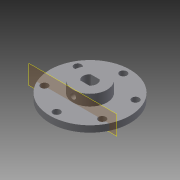
# Autodesk Inventor part: Snowblower Hub
Saved by Autodesk Inventor 2014 (Build 180170000, 170)
## iProperties
Created: 2014-01-06
Part Number: Snowblower Hub
Material: Generic
Document SubType Name: Modeling
Designer: Andrew Toennies
Density: 1 g/cm^3
Appearance: Default
Author: Andrew Toennies
Autodesk Inventor part; units mm, degrees
ref_plane "YZ Plane" through (0, 0, 0) normal (1, 0, 0) x (0, 1, 0)
ref_plane "XZ Plane" through (0, 0, 0) normal (0, 1, 0) x (-1, 0, 0)
ref_plane "XY Plane" through (0, 0, 0) normal (0, 0, 1) x (1, 0, 0)
sketch "Sketch1" plane through (0, 0, 0) normal (0, 1, 0) x (-1, 0, 0)
  circle A0 centre (0, 0) radius 28.575
  dimension "d0" = 57.15
  constraints: 1 centre point, 1 coincident
  measures "d0" diameter of A0
extrude "Extrusion1" add sketch "Sketch1" along normal blind 4.572
sketch "Sketch2" plane through (0, 4.572, 0) normal (0, 1, 0) x (1, 0, 0)
  circle A0 centre (0, 0) radius 28.575 projected
  circle A1 centre (0, 0) radius 12.1666
  dimension "d3" = 24.3332
  constraints: 1 centre point, 1 coincident
  measures "d3" diameter of A1
extrude "Extrusion2" add sketch "Sketch2" along normal blind 7.874 contours A1
sketch "Sketch3" plane through (0, 4.572, 0) normal (0, 1, 0) x (1, 0, 0)
  circle A0 centre (0, 0) radius 28.575 projected
  circle A1 centre (0, 0) radius 23.8125 construction
  circle A2 centre (0, 23.8125) radius 2.5908
  line L0 (0, 0) -> (0, 23.8125) construction
  circle A3 centre (-20.6222, 11.9063) radius 2.5908
  circle A4 centre (-20.6222, -11.9062) radius 2.5908
  circle A5 centre (0, -23.8125) radius 2.5908
  circle A6 centre (20.6222, -11.9063) radius 2.5908
  circle A7 centre (20.6222, 11.9062) radius 2.5908
  dimension "d6" = 47.625
  dimension "d7" = 5.1816
  dimension "d10" = 360
  constraints: 6 centre point, 2 end point, 1 coincident, 1 vertical, 1 vertical alignment, 15 other
  measures "d7" diameter of A2
extrude "Extrusion3" cut sketch "Sketch3" against normal blind 7.874 contours A2 | A3 | A4 | A5 | A6 | A7
sketch "Sketch4" plane through (0, 12.446, 0) normal (0, 1, 0) x (1, 0, 0)
  circle A0 centre (0, 0) radius 12.1666 projected
  line L0 (-3.304, 3.7529) -> (3.304, 3.7529)
  line L1 (-3.304, -3.7528) -> (3.304, -3.7528)
  line L2 (3.304, 3.7529) -> (3.304, -3.7528) construction
  line L3 (-3.304, 3.7529) -> (-3.304, -3.7528) construction
  arc A1 (-3.304, 3.7529) -> (-3.304, -3.7528) centre (0, 0) ccw
  arc A2 (3.304, -3.7528) -> (3.304, 3.7529) centre (0, 0) ccw
  dimension "d15" = 7.5057
  dimension "d16" = 5
  dimension "d17" = 5
  constraints: 8 end point, 4 point on circle, 2 centre point, 2 parallel, 1 coincident, 1 horizontal, 1 perpendicular
  measures "d15" distance between parallel lines of L0 L1
  measures "d16" radius of A2
  measures "d17" radius of A1
extrude "Extrusion4" cut sketch "Sketch4" against normal blind 14.986 contours L0 A2 L1 A1
ref_plane "Work Plane1" through (0, 4.572, 12.1666) normal (0, 0, 1) x (1, 0, 0)
sketch "Sketch5" plane through (0, 4.572, 12.1666) normal (0, 0, 1) x (1, 0, 0)
  circle A0 centre (0, 3.937) radius 2.0193
  line L0 (0, -4.572) -> (0, 3.937) construction
  line L1 (-28.575, -4.572) -> (28.575, -4.572) construction
  dimension "d20" = 8.509
  dimension "d21" = 4.0386
  constraints: 2 end point, 1 centre point, 1 vertical
  measures "d20" distance from line of L1 L0.end
  measures "d21" diameter of A0
extrude "Extrusion5" cut sketch "Sketch5" against normal blind 12.3698
body "Solid1"
